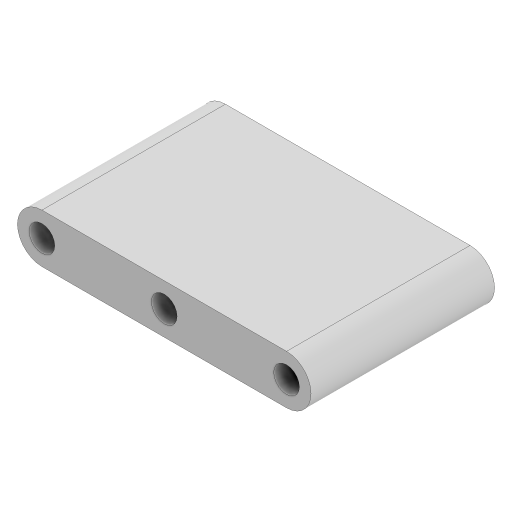
# Autodesk Inventor part: battery_top_secure
Saved by Autodesk Inventor 2023 (Build 270158000, 158)
## iProperties
Created: 2024-05-15
Part Number: battery_top_secure
Material: Generic
Document SubType Name: Modeling
Designer: Thomas
Density: 1 g/cm^3
Appearance: Default
Author: Thomas
Autodesk Inventor part; units mm, degrees
ref_plane "YZ Plane" through (0, 0, 0) normal (1, 0, 0) x (0, 1, 0)
ref_plane "XZ Plane" through (0, 0, 0) normal (0, 1, 0) x (-1, 0, 0)
ref_plane "XY Plane" through (0, 0, 0) normal (0, 0, 1) x (1, 0, 0)
sketch "Sketch1" plane through (0, 0, 0) normal (0, 0, 1) x (1, 0, 0)
  circle A0 centre (0, 0) radius 2.1
  circle A1 centre (20, 0) radius 2.1
  circle A2 centre (40, 0) radius 2.1
  line L0 (0, 0) -> (40, 0) construction
  line L1 (0, 0) -> (40, 0) construction
  line L2 (0, -4) -> (40, -4)
  line L3 (40, 4) -> (0, 4)
  arc A3 (0, 4) -> (0, -4) centre (0, 0) ccw
  arc A4 (40, -4) -> (40, 4) centre (40, 0) ccw
  dimension "d0" = 4.2
  dimension "d1" = 4.2
  dimension "d2" = 4.2
  dimension "d3" = 20
  dimension "d4" = 20
  dimension "d5" = 0
  dimension "d6" = 8
  constraints: 10 end point, 5 centre point, 4 point on circle, 4 tangent, 2 equal length, 1 coincident, 1 horizontal, 1 midpoint
  measures "d0" diameter of A0
  measures "d1" diameter of A1
  measures "d2" diameter of A2
  measures "d3" distance of point (0, 0) A1.centre
  measures "d4" distance of L0.end A1.centre
  measures "d5" distance from line of A1.centre L0
  measures "d6" diameter of A4
extrude "Extrusion1" add sketch "Sketch1" against normal blind 30
body "Solid1"
